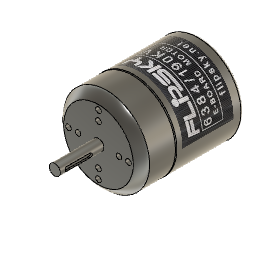
FlipskyR6374 v1 (Autodesk Fusion 360 design; units mm, degrees)
Autodesk Fusion 360 part; units mm, degrees
note: some values were not read from the file. Set by a fixed rule: which sketch regions a step uses.
sketch "FlipskyFrontSketch" plane through (0, 0, 0) normal (0, 1, 0) x (1, 0, 0) in component "FlipskyR6374"
  circle A0 centre (0, 0) radius 22 construction
  circle A1 centre (0, 0) radius 31.5
  circle A2 centre (0, 0) radius 15 construction
  circle A3 centre (0, 0) radius 4
  line L0 (0, -40.5211) -> (0, 42) construction
  line L1 (-68.5254, 0) -> (76.0881, 0) construction
  circle A4 centre (0, -22) radius 2
  circle A5 centre (0, -15) radius 2
  circle A6 centre (0, 22) radius 2
  circle A7 centre (0, 15) radius 2
  circle A8 centre (-15, 0) radius 2
  circle A9 centre (-22, 0) radius 2
  circle A10 centre (15, 0) radius 2
  circle A11 centre (22, 0) radius 2
  line L2 (3.7081, -1.5) -> (2.5, -1.5)
  line L3 (2.5, -1.5) -> (2.5, 1.5)
  line L4 (2.5, 1.5) -> (3.7081, 1.5)
  line L5 (60, 20) -> (60, -20)
  line L6 (-60, -20) -> (-60, 20)
  line L7 (-60, 20) -> (60, -20) construction
  line L8 (60, 20) -> (-60, -20) construction
  line L9 (-28.1114, -20) -> (-60, -20)
  line L10 (60, -20) -> (28.1114, -20)
  line L11 (-60, 20) -> (-28.1114, 20)
  line L12 (28.1114, 20) -> (60, 20)
  circle A12 centre (-50, -10) radius 2.5
  circle A13 centre (-50, 10) radius 2.5
  circle A14 centre (50, -10) radius 2.5
  circle A15 centre (50, 10) radius 2.5
  line L13 (-63.5493, -10) -> (64.0522, -10) construction
  line L14 (-62.7711, 10) -> (65, 10) construction
  line L15 (-50, -26.3815) -> (-50, 24.1685) construction
  line L16 (50, -27.289) -> (50, 25) construction
  line L17 (16.7321, 1) -> (14.9666, 1)
  line L18 (2.5, -1) -> (3, -1)
  line L19 (-40, -20) -> (-40, 20)
  line L20 (40, -20) -> (40, 20)
  arc A16 (-28.1114, -20) -> (28.1114, -20) centre (0, 0) ccw
  arc A17 (28.1114, 20) -> (-28.1114, 20) centre (0, 0) ccw
  circle A18 centre (0, 0) radius 10
  circle A19 centre (0, 0) radius 5
  line L21 (0, 0) -> (-31.8198, -31.8198) construction
  line L22 (0, 0) -> (45, 0) construction
  line L23 (-16.2768, -30.419) -> (-14.0506, -28.1927)
  line L24 (-34.1421, -20) -> (-28.1927, -14.0506)
  dimension "d1" = 44
  dimension "d2" = 63
  dimension "d3" = 30
  dimension "d4" = 8
  dimension "d6" = 4
  dimension "d7" = 4
  dimension "d8" = 4
  dimension "d9" = 4
  dimension "d10" = 4
  dimension "d11" = 4
  dimension "d12" = 4
  dimension "d13" = 4
  dimension "d28" = 1.5
  dimension "d29" = 1.5
  dimension "d30" = 2.5
  dimension "d35" = 120
  dimension "d36" = 40
  dimension "d48" = 5
  dimension "d49" = 5
  dimension "d50" = 5
  dimension "d51" = 5
  dimension "d52" = 10
  dimension "d53" = 10
  dimension "d54" = 10
  dimension "d55" = 10
  dimension "d66" = 20
  dimension "d67" = 20
  dimension "d68" = 34.5
  dimension "d71" = 20
  dimension "d72" = 10
  dimension "d73" = 135
  dimension "d75" = 10
  dimension "d76" = 10
  constraint coincident A0.centre A1.centre
  constraint concentric A0 A3
  constraint vertical L0
  constraint horizontal L1
  constraint coincident A0.centre L0
  constraint coincident A0.centre L1
  constraint coincident A0 A4.centre
  constraint coincident L0 A4.centre
  constraint coincident A2 A5.centre
  constraint coincident L0 A5.centre
  constraint coincident A0 A6.centre
  constraint coincident L0 A6.centre
  constraint coincident A2 A7.centre
  constraint coincident L0 A7.centre
  constraint coincident L1 A8.centre
  constraint coincident A2 A8.centre
  constraint coincident A0 A9.centre
  constraint coincident L1 A9.centre
  constraint coincident L1 A10.centre
  constraint coincident A2 A10.centre
  constraint coincident A0 A11.centre
  constraint coincident L1 A11.centre
  constraint horizontal L2
  constraint vertical L3
  constraint horizontal L4
  constraint coincident A3 L4.end
  constraint coincident A3 L2.start
  constraint horizontal L11
  constraint perpendicular L5 L11
  constraint parallel L10 L11
  constraint parallel L5 L6
  constraint coincident L7 A0.centre
  constraint coincident L8 A0.centre
  constraint collinear L9 L10
  constraint collinear L11 L12
  constraint concentric A2 A16
  constraint coincident L12.start A16
  constraint perpendicular L5 L13
  constraint perpendicular L5 L14
  constraint perpendicular L12 L16
  constraint coincident A12.centre L13
  constraint coincident A12.centre L15
  constraint coincident A13.centre L15
  constraint coincident A13.centre L14
  constraint coincident A15.centre L14
  constraint coincident A15.centre L16
  constraint coincident A14.centre L13
  constraint coincident A14.centre L16
  constraint vertical L15
  constraint coincident A2 L17.end
  constraint coincident A10 L17.start
  constraint coincident L3 L18.start
  constraint coincident L7 L18.end
  constraint coincident L9 L19.start
  constraint coincident L11 L19.end
  constraint perpendicular L11 L19
  constraint coincident L10 L20.start
  constraint coincident L12 L20.end
  constraint perpendicular L12 L20
  constraint concentric A16 A17
  constraint concentric A1 A19
  constraint horizontal L22
  constraint parallel L21 L23
  constraint parallel L21 L24
  constraint coincident A1 L24.end
  constraint coincident A1 L23.end
  constraint coincident A16 L23.start
  constraint coincident L9 L24.start
  measures "d1" diameter of A0
  measures "d2" diameter of A1
  measures "d3" diameter of A2
  measures "d4" diameter of A3
  measures "d6" diameter of A4
  measures "d7" diameter of A5
  measures "d8" diameter of A6
  measures "d9" diameter of A7
  measures "d10" diameter of A8
  measures "d11" diameter of A9
  measures "d12" diameter of A10
  measures "d13" diameter of A11
  measures "d28" distance of L1 L2
  measures "d29" distance of L1 L4
  measures "d30" distance of A0.centre L3
  measures "d35" distance of L5.end L6.start
  measures "d36" distance of L5.start L5.end
  measures "d48" diameter of A12
  measures "d49" diameter of A13
  measures "d50" diameter of A14
  measures "d51" diameter of A15
  measures "d52" distance of L9 L13
  measures "d53" distance of L11 L14
  measures "d54" distance of L6 A12.centre
  measures "d55" distance of L5 L16
  measures "d66" distance of L6 L19
  measures "d67" distance of L5 L20
  measures "d68" radius of A16
  measures "d71" diameter of A18
  measures "d72" diameter of A19
  measures "d73" angle of L21 L22
  measures "d75" distance of L21 L23
  measures "d76" distance of L21 L24
extrude "Extrude1" add sketch "FlipskyFrontSketch" along normal blind 25 contours A1 | A4 | A5 | A6 | A7 | A8 | A9 | A10 | A11 | A18 | A19 makes body 1 in component "Stator"
extrude "Extrude2" cut sketch "FlipskyFrontSketch" along normal blind 5 contours A4 | A5 | A6 | A7 | A8 | A9 | A10 | A11 bodies 1 in component "Stator"
fillet "Fillet1" radius 6 tangency weight 0.2 1 edges at (-29.3683, 0, 11.3909) on bodies 1 in component "Stator"
sketch "AxleRightSketch" plane through (0, 0, 0) normal (1, 0, 0) x (0, 1, 0) in component "Rotor"
  line L0 (-27, 1.5) -> (-10, 1.5)
  line L1 (-10, -1.5) -> (-27, -1.5)
  line L2 (-35, 0) -> (6.0427, 0) construction
  line L3 (-32, 10) -> (-32, -10) construction
  line L4 (0, -20) -> (0, 20)
  arc A0 (-27, 1.5) -> (-27, -1.5) centre (-27, 0) ccw
  arc A1 (-10, -1.5) -> (-10, 1.5) centre (-10, 0) ccw
  dimension "d92" = 3
  dimension "d93" = 3
  dimension "d94" = 17
  dimension "d95" = 10
  constraint tangent L0 A1
  constraint tangent L0 A0
  constraint horizontal L2
  constraint coincident L2 origin
  constraint coincident A1.centre L2
  constraint coincident A0.centre L2
  constraint tangent L1 A1
  constraint tangent L1 A0
  constraint vertical L3
  measures "d92" diameter of A0
  measures "d93" diameter of A1
  measures "d94" distance of A0.centre A1.centre
  measures "d95" distance of A1.centre origin
extrude "Extrude1'" add sketch "FlipskyFrontSketch" along normal blind -32 and the other way blind -74 separate body contours A3 L2 L3 L4 | A3 L2 L3 L4 makes body 2 in component "Rotor"
extrude "Extrude5" add sketch "FlipskyFrontSketch" along normal blind 75 and the other way blind -26 contours A1 | A3 L2 L3 L4 | A3 L2 L3 L4 | A4 | A5 | A6 | A7 | A8 | A9 | A10 | A11 | A18 | A19 bodies 2 in component "Rotor"
fillet "Fillet1'" radius 2 1 edges at (-29.3683, 75, 11.3909) on bodies 2 in component "Rotor"
extrude "Extrude2'" cut sketch "AxleRightSketch" along normal blind 15 and the other way blind -2.5 bodies 2 in component "Rotor"
component "FlipskyR6374" placed x (1, 0, 0) y (0, 1, 0) z (0, 0, 1) at (0, 0, 0)
component "Flipsky6374" placed x (1, 0, 0) y (0, 1, 0) z (0, 0, 1) at (0, 0, 0) in component "FlipskyR6374"
component "Stator" placed x (1, 0, 0) y (0, 1, 0) z (0, 0, 1) at (0, 0, 0) in component "Flipsky6374"
component "Rotor" placed x (1, 0, 0) y (0, 1, 0) z (0, 0, 1) at (0, 0, 0) in component "Flipsky6374"
